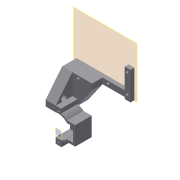
# Autodesk Inventor part: cellSTORM_v5_focusmotormount
Saved by Autodesk Inventor 2019 (Build 230136000, 136)
## iProperties
Created: 2020-05-04
Part Number: cellSTORM_v5_focusmotormount
Material: Generic
Document SubType Name: Modeling
Designer: diederichbenedict
Density: 1 g/cm^3
Appearance: Default
Author: diederichbenedict
Autodesk Inventor part; units mm, degrees
ref_plane "YZ Plane" through (0, 0, 0) normal (1, 0, 0) x (0, 1, 0)
ref_plane "XZ Plane" through (0, 0, 0) normal (0, 1, 0) x (-1, 0, 0)
ref_plane "XY Plane" through (0, 0, 0) normal (0, 0, 1) x (1, 0, 0)
ref_plane "Work Plane1" through (0, 0, 0) normal (0, 0, 1) x (1, 0, 0)
sketch "Sketch1" plane through (0, 0, 0) normal (0, 0, 1) x (1, 0, 0)
  line L0 (-45, 22) -> (22, 22) projected
  line L1 (22, 22) -> (22, -22) projected
  line L2 (22, -22) -> (-45, -22) projected
  line L3 (-45, -28) -> (-45, -22) projected
  line L4 (-30, -28) -> (-45, -28) projected
  line L5 (-30, -28) -> (-28, -30) projected
  line L6 (-28, -30) -> (28, -30) projected
  line L7 (28, -30) -> (30, -28) projected
  line L8 (30, -28) -> (30, 28) projected
  line L9 (30, 28) -> (28, 30) projected
  line L10 (28, 30) -> (-28, 30) projected
  line L11 (-28, 30) -> (-30, 28) projected
  line L12 (-30, 28) -> (-45, 28) projected
  line L13 (-45, 22) -> (-45, 28) projected
  circle A0 centre (25, 25) radius 1.95 projected
  circle A1 centre (25, 0) radius 1.95 projected
  circle A2 centre (0, 25) radius 1.95 projected
  circle A3 centre (-25, -25) radius 1.95 projected
  circle A4 centre (25, -25) radius 1.95 projected
  circle A5 centre (-25, 25) radius 1.95 projected
  circle A6 centre (0, -25) radius 1.95 projected
  line L14 (30, 4.1832) -> (22.5, 4.1832)
  line L15 (22.5, 4.1832) -> (22.5, -32.3594)
  line L16 (22.5, -32.3594) -> (30, -32.3594)
  line L17 (30, -32.3594) -> (30, 4.1832)
  line L18 (22.5, -22.5) -> (-45, -22.5)
  line L19 (-45, -22.5) -> (-45, -30)
  line L20 (-45, -30) -> (22.5, -30)
  line L21 (22.5, -30) -> (22.5, -22.5)
  circle A7 centre (25, 0) radius 2.15
  circle A8 centre (25, -25) radius 2.15
  circle A9 centre (0, -25) radius 2.15
  circle A10 centre (-25, -25) radius 2.15
  point P0 (0, 0)
  dimension "d0" = 0
  dimension "d1" = 0.5
  dimension "d2" = 0.5
  dimension "d3" = 0.2
  dimension "d4" = 0.2
  dimension "d5" = 0.2
  dimension "d6" = 0.2
  constraints: 16 end point, 4 centre point, 4 parallel, 3 point on line, 2 horizontal, 2 perpendicular
  measures "d0" distance between parallel lines of L8 L17
  measures "d1" distance between parallel lines of L1 L15
  measures "d2" distance between parallel lines of L2 L18
  measures "d3" radial gap between concentric circles of A1 A7
  measures "d4" radial gap between concentric circles of A4 A8
  measures "d5" radial gap between concentric circles of A6 A9
  measures "d6" radial gap between concentric circles of A3 A10
extrude "Extrusion1" add sketch "Sketch1" along normal blind 5 contours L18 L15 L6 L5 L4 L3 | L4 L5 L20 L19 | L15 L14 L8 L7 L6 | L6 L7 L17 L16 L15
ref_plane "Work Plane2" through (-32, -78.0277, 40.0715) normal (0, 0, -1) x (0, 1, 0)
sketch "Sketch2" plane through (-32, -78.0277, 40.0715) normal (0, 0, -1) x (0, 1, 0)
  arc A0 (-8.1223, 3.5) -> (-12.3223, 3.5) centre (-10.2223, 3.5) ccw projected
  arc A1 (-1.4723, 14.4287) -> (-6.2777, 7) centre (7.2777, 3.5) ccw projected
  arc A2 (20.8332, 7) -> (16.0277, 14.4287) centre (7.2777, 3.5) ccw projected
  arc A3 (22.6777, 3.5) -> (26.8777, 3.5) centre (24.7777, 3.5) ccw projected
  line L0 (-6.2777, 0) -> (-10.2223, 0) projected
  arc A4 (-6.7223, 3.5) -> (21.2777, 3.5) centre (7.2777, 3.5) ccw projected
  line L1 (-6.5873, 0) -> (-14.2223, 0)
  line L2 (-14.2223, 0) -> (-14.2223, 7.5835)
  line L3 (-14.2223, 7.5835) -> (-8.5689, 7.5835)
  line L4 (21.1796, 0.1492) -> (27.0132, 0.1492)
  line L5 (27.0132, 0.1492) -> (28.7777, 0.1492)
  line L6 (28.7777, 0.1492) -> (28.7777, 7.1168)
  line L7 (28.7777, 7.1168) -> (23.2373, 7.1168)
  circle A5 centre (24.7777, 3.5) radius 1.4
  circle A6 centre (-10.2223, 3.5) radius 1.4
  line L8 (-1.7723, 14.5719) -> (-4.7723, 14.5719)
  line L9 (-4.7723, 14.5719) -> (-4.7723, 25.3)
  line L10 (-4.7723, 25.3) -> (-1.7723, 25.3)
  line L11 (-1.7723, 25.3) -> (-1.7723, 14.5719)
  line L12 (16.3277, 14.5719) -> (19.3277, 14.5719)
  line L13 (19.3277, 14.5719) -> (19.3277, 25.3)
  line L14 (19.3277, 25.3) -> (16.3277, 25.3)
  line L15 (16.3277, 25.3) -> (16.3277, 14.5719)
  line L16 (16.3277, 25.3) -> (-1.7723, 25.3)
  line L17 (-1.7723, 25.3) -> (-1.7723, 22.3)
  line L18 (-1.7723, 22.3) -> (16.3277, 22.3)
  line L19 (16.3277, 22.3) -> (16.3277, 25.3)
  arc A7 (21.1796, 0.1492) -> (16.3277, 14.5719) centre (7.2777, 3.5) ccw
  arc A8 (-1.7723, 14.5719) -> (-6.5873, 0) centre (7.2777, 3.5) ccw
  arc A9 (23.2373, 7.1168) -> (19.3277, 14.5719) centre (7.2777, 3.5) ccw
  arc A10 (-4.7723, 14.5719) -> (-8.5689, 7.5835) centre (7.2777, 3.5) ccw
  line L20 (-1.4723, 22) -> (16.0277, 22)
  point P0 (78.0277, 32)
  dimension "d14" = 2.8
  dimension "d15" = 2.8
  dimension "d16" = 4
  dimension "d17" = 4
  dimension "d33" = 3
  dimension "d36" = 3
  dimension "d37" = 3
  dimension "d40" = 0.3
  dimension "d41" = 0.3
  dimension "d42" = 0.3
  dimension "d43" = 0.3
  dimension "d44" = 0.3
  constraints: 40 end point, 8 point on circle, 7 perpendicular, 6 centre point, 6 horizontal, 6 parallel, 4 coincident, 3 point on line, 4 other
  measures "d14" diameter of A5
  measures "d15" diameter of A6
  measures "d16" distance from line of L2 A0.centre
  measures "d17" distance from line of L6 A3.centre
  measures "d33" distance of L10.end L9.end
  measures "d36" distance of L14.end L13.end
  measures "d37" distance between parallel lines of L18 L16
  measures "d40" distance from line of L15 A2.end
  measures "d41" distance between parallel lines of L20 L18
  measures "d42" distance from line of A1.start L11
  measures "d43" radial gap between concentric circles of A1 A8
  measures "d44" radial gap between concentric circles of A2 A7
ref_plane "Work Plane3" through (-42.5, -74.75, 21.5715) normal (0, 0, -1) x (0, 1, 0)
extrude "Extrusion2" add sketch "Sketch2" along normal up to surface (18.5 mm away)
sketch "Sketch3" plane through (-24.8832, -49.25, 21.5715) normal (0, 0, -1) x (-1, 0, 0)
  arc A0 (6.9676, -7.5981) -> (-7.4551, -12.45) centre (3.6168, -21.5) ccw projected
  line L0 (6.9676, 0) -> (6.9676, -7.5981) projected
  line L1 (0, 0) -> (6.9676, 0) projected
  line L2 (0, -5.5404) -> (0, 0) projected
  arc A1 (0, -5.5404) -> (-7.4551, -9.45) centre (3.6168, -21.5) ccw projected
  circle A2 centre (3.6168, -4) radius 1.4 projected
  arc A3 (6.9676, -7.5981) -> (-7.4551, -12.45) centre (3.6168, -21.5) ccw projected
  line L3 (-18.1832, -9.45) -> (-7.4551, -9.45) projected
  line L4 (-15.1832, -12.45) -> (-15.1832, -30.55) projected
  line L5 (-7.4551, -12.45) -> (-15.1832, -12.45) projected
  line L6 (-18.1832, -33.55) -> (-18.1832, -9.45) projected
  line L7 (-7.4551, -33.55) -> (-18.1832, -33.55) projected
  arc A4 (-7.4551, -33.55) -> (-0.4667, -37.3466) centre (3.6168, -21.5) ccw projected
  line L8 (-0.4667, -43) -> (-0.4667, -37.3466) projected
  line L9 (7.1168, -43) -> (-0.4667, -43) projected
  line L10 (7.1168, -35.3651) -> (7.1168, -43) projected
  arc A5 (-7.4551, -30.55) -> (7.1168, -35.3651) centre (3.6168, -21.5) ccw projected
  line L11 (-15.1832, -30.55) -> (-7.4551, -30.55) projected
  line L12 (7.1168, -35.3651) -> (6.9676, -7.5981)
  point P0 (-24.8832, 49.25)
  point P1 (7.3934, -35.5712)
  constraints: 2 end point, 1 other
extrude "Extrusion3" add sketch "Sketch3" along normal blind 3 contours L12 A5 L11 L4 L5 A0 | A0 L5 L4 L11 A5 L10 L9 L8 A4 L7 L6 L3 A1 L2 L1 L0 | A2
sketch "Sketch4" plane through (0, 0, 5) normal (0, 0, 1) x (1, 0, 0)
  circle A0 centre (25, 0) radius 2.15 projected
  circle A1 centre (25, -25) radius 2.15 projected
  circle A2 centre (-25, -25) radius 2.15 projected
  circle A3 centre (0, -25) radius 2.15 projected
  line L0 (22.5, -22.5) -> (-45, -22.5) projected
  line L1 (-45, -22.5) -> (-45, -30) projected
  line L2 (-45, -30) -> (22.5, -30) projected
  line L3 (22.5, -30) -> (22.5, -32.3594) projected
  line L4 (22.5, -32.3594) -> (30, -32.3594) projected
  line L5 (30, -32.3594) -> (30, 4.1832) projected
  line L6 (30, 4.1832) -> (22.5, 4.1832) projected
  line L7 (22.5, 4.1832) -> (22.5, -22.5) projected
  arc A4 (-25, -57.1946) -> (-32, -57.1946) centre (-28.5, -70.75) ccw projected
  line L8 (-45, -22.5) -> (-45, -30) projected
  arc A5 (-17.4281, -61.7) -> (-31.8508, -56.8481) centre (-28.5, -70.75) ccw projected
  line L9 (-45, -22.5) -> (-31.8508, -22.5)
  line L10 (-31.8508, -22.5) -> (-31.8508, -56.8481)
  line L11 (-31.8508, -56.8481) -> (-45, -56.8481)
  line L12 (-45, -56.8481) -> (-45, -22.5)
  line L13 (-25, -56.8849) -> (-6.175, -30)
  line L14 (-45, -30) -> (22.5, -30) projected
  line L15 (-25, -56.8849) -> (7.8204, -56.8849) construction
  line L16 (-6.175, -30) -> (-6.175, -22.5)
  line L17 (22.5, -22.5) -> (-45, -22.5) projected
  line L18 (-25, -53.25) -> (-25, -57.1946) projected
  line L19 (-31.8508, -22.5) -> (-6.175, -22.5)
  line L20 (-6.175, -22.5) -> (-6.175, -30)
  line L21 (-6.175, -30) -> (-31.8508, -30)
  line L22 (-31.8508, -30) -> (-31.8508, -22.5)
  point P0 (0, 0)
  point P1 (-32, -84.6151)
  dimension "d20" = 55
  constraints: 22 end point, 4 parallel, 3 horizontal, 3 perpendicular, 3 point on line, 1 equal length, 1 point on circle
  measures "d20" angle of L15 L13
extrude "Extrusion4" add sketch "Sketch4" along normal up to surface (13.5715 mm away) contours L16 L2 L10 L0 | L10 L2 L1 L0 | L13 A5 L10 L2 | L10 L11 L12 L2
sketch "Sketch5" plane through (-45, -30, 0) normal (-1, 0, 0) x (0, 0, 1)
  line L0 (40.0715, -26.8481) -> (40.0715, -19.25) projected
  line L1 (40.0715, -19.25) -> (18.5715, -19.25) projected
  line L2 (18.5715, -26.8481) -> (18.5715, 7.5) projected
  line L3 (40.0715, -26.8481) -> (40.0715, -19.25) projected
  line L4 (0, 7.5) -> (18.5715, 7.5) projected
  line L5 (40.0715, -19.25) -> (18.5715, 7.5)
  line L6 (40.0715, -26.8481) -> (21.5715, -26.8481) projected
  line L7 (21.5715, -26.8481) -> (18.5715, -26.8481) projected
  line L8 (18.5715, -26.8481) -> (18.5715, -19.25) projected
  line L9 (40.0715, -19.25) -> (18.5715, -19.25)
  line L10 (18.5715, -19.25) -> (18.5715, 7.5)
  line L11 (18.5715, 7.5) -> (40.0715, -19.25)
  line L12 (40.0715, -19.25) -> (18.5715, -19.25)
  line L13 (18.5715, -19.25) -> (18.5715, -26.8481)
  line L14 (18.5715, -26.8481) -> (40.0715, -26.8481)
  line L15 (40.0715, -26.8481) -> (40.0715, -19.25)
  point P0 (0, 30)
  point P1 (5, 7.5)
  constraints: 16 end point, 4 equal length, 2 perpendicular, 1 horizontal
extrude "Extrusion5" add sketch "Sketch5" against normal up to surface (13.1492 mm away)
sketch "Sketch6" plane through (-31.8508, -49.25, 18.5715) normal (1, 0, 0) x (0, 0, -1)
  line L0 (-21.5, 0) -> (0, 0) projected
  line L1 (0, 26.75) -> (0, 0) projected
  circle A0 centre (-10.75, 3.0956) radius 1.4
  line L2 (0, 26.75) -> (-21.5, 0) projected
  point P0 (18.5715, 49.25)
  dimension "d25" = 2.8
  constraints: 1 centre point
  measures "d25" diameter of A0
hole "Hole1" at (-31.8508, -46.1544, 29.3215) direction (-1, 0, 0) diameter 2.8 depth 20 tip angle 118 counterbore diameter 7.5 counterbore depth 4.775
body "Solid1"
